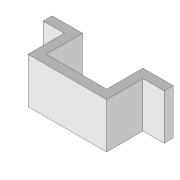
# Autodesk Inventor part: Staender
Saved by Autodesk Inventor 2020 (Build 240168000, 168)
## iProperties
Created: 2020-03-18
Part Number: Staender
Material: Generisch
Document SubType Name: Modeling
Designer: franz
Density: 1 g/cm^3
Appearance: Vorgabe
Author: franz
Autodesk Inventor part; units mm, degrees
ref_plane "YZ Plane" through (0, 0, 0) normal (1, 0, 0) x (0, 1, 0)
ref_plane "XZ Plane" through (0, 0, 0) normal (0, 1, 0) x (-1, 0, 0)
ref_plane "XY Plane" through (0, 0, 0) normal (0, 0, 1) x (1, 0, 0)
sketch "Skizze1" plane through (0, 0, 0) normal (0, 1, 0) x (-1, 0, 0)
  line L0 (200, -150) -> (100, -150)
  line L1 (100, -150) -> (100, -30)
  line L2 (100, -30) -> (-100, -30)
  line L3 (-100, -30) -> (-100, -150)
  line L4 (-100, -150) -> (-200, -150)
  line L5 (-200, -150) -> (-200, -120)
  line L6 (-200, -120) -> (-130, -120)
  line L7 (-130, -120) -> (-130, 0)
  line L8 (-130, 0) -> (130, 0)
  line L9 (130, 0) -> (130, -120)
  line L10 (130, -120) -> (200, -120)
  line L11 (200, -120) -> (200, -150)
  line L12 (0, -180) -> (0, 30) projected
  point P0 (0, 0)
  dimension "d0" = 30
  dimension "d1" = 30
  dimension "d3" = 30
  dimension "d4" = 200
  dimension "d5" = 100
  dimension "d6" = 150
  constraints: 24 end point, 10 perpendicular, 1 horizontal, 1 midpoint, 5 other
  measures "d0" distance of L10.end L0.start
  measures "d1" distance between parallel lines of L1 L9
  measures "d3" distance between parallel lines of L8 L2
  measures "d4" distance of L1.end L2.end
  measures "d5" distance between parallel lines of L1 L11
  measures "d6" distance between parallel lines of L8 L4
extrude "Extrusion1" add sketch "Skizze1" along normal blind 150
sketch "Skizze2" plane through (-130, 0, 0) normal (0, 0, 1) x (1, 0, 0)
  line L0 (230, 0) -> (30, 0) projected
  line L1 (55, 30) -> (205, 30)
  line L2 (205, 30) -> (205, 0)
  line L3 (205, 0) -> (55, 0)
  line L4 (55, 0) -> (55, 30)
  line L5 (260, 0) -> (260, 150) projected
  line L6 (0, 0) -> (0, 150) projected
  point P0 (130, 0)
  dimension "d9" = 260
  dimension "d10" = 30
  dimension "d11" = 150
  dimension "d12" = 55
  constraints: 8 end point, 2 parallel, 1 horizontal, 1 perpendicular, 1 point on line
  measures "d9" distance between parallel lines of L5 L6
  measures "d10" distance of L1.end L2.end
  measures "d11" distance of L1.start L1.end
  measures "d12" distance between parallel lines of L6 L4
extrude "Extrusion2" add sketch "Skizze2" along normal blind 300
sketch "Skizze3" plane through (0, 0, 0) normal (0, -1, 0) x (1, 0, 0)
  line L0 (-75, 300) -> (75, 300) projected
  line L1 (75, 0) -> (75, 300) projected
  line L2 (-75, 300) -> (75, 300)
  line L3 (75, 300) -> (75, 270)
  line L4 (75, 270) -> (-75, 270)
  line L5 (-75, 270) -> (-75, 300)
  point P0 (0, 0)
  dimension "d15" = 30
  constraints: 8 end point, 2 parallel, 1 horizontal, 1 perpendicular, 1 point on line
  measures "d15" distance of L2.end L3.end
extrude "Extrusion3" add sketch "Skizze3" along normal blind 400
sketch "Skizze4" plane through (-130, 0, 300) normal (0, 0, 1) x (1, 0, 0)
  line L0 (110, -355) -> (150, -355)
  line L1 (150, -355) -> (150, -335)
  line L2 (150, -335) -> (110, -335)
  line L3 (110, -335) -> (110, -355)
  line L4 (110, -355) -> (150, -335) construction
  line L5 (150, -355) -> (110, -335) construction
  point P0 (130, 0)
  point P1 (130, -345)
  dimension "d18" = 40
  dimension "d19" = 20
  dimension "d20" = 345
  dimension "d21" = 0
  constraints: 12 end point, 2 midpoint, 2 parallel, 1 horizontal, 1 perpendicular
  measures "d18" distance of L2.end L1.end
  measures "d19" distance of L1.end L0.end
  measures "d20" distance of point (130, -345) point (130, 0)
  measures "d21" horizontal distance of point (130, -345) point (130, 0)
extrude "Extrusion4" cut sketch "Skizze4" against normal through all
equation "\"d1\" = d0"
equation "\"d3\" = d0"
equation "\"d12\" = -0.5 * d11 + 0.5 * d9"
